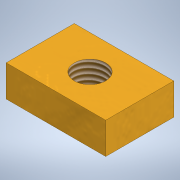
# Autodesk Inventor part: Part26
Saved by Autodesk Inventor 2020 (Build 240168000, 168)
## iProperties
Created: 2021-10-14
Part Number: Part26
Material: Brass, Soft Yellow, Welded
Document SubType Name: Modeling
Designer: simon.erikssonwestl
Density: 8.5 g/cm^3
Appearance: Weld - Brass
Author: simon.erikssonwestl
Autodesk Inventor part; units mm, degrees
ref_plane "YZ Plane" through (0, 0, 0) normal (1, 0, 0) x (0, 1, 0)
ref_plane "XZ Plane" through (0, 0, 0) normal (0, 1, 0) x (-1, 0, 0)
ref_plane "XY Plane" through (0, 0, 0) normal (0, 0, 1) x (1, 0, 0)
sketch "Sketch1" plane through (0, 0, 0) normal (0, 1, 0) x (-1, 0, 0)
  line L0 (4.75, 3.25) -> (-4.75, 3.25)
  line L1 (-4.75, 3.25) -> (-4.75, -3.25)
  line L2 (-4.75, -3.25) -> (4.75, -3.25)
  line L3 (4.75, -3.25) -> (4.75, 3.25)
  line L4 (4.75, 3.25) -> (-4.75, -3.25) construction
  line L5 (-4.75, 3.25) -> (4.75, -3.25) construction
  circle A0 centre (0, 0) radius 1.5
  dimension "d0" = 9.5
  dimension "d1" = 6.5
  dimension "d2" = 3
  constraints: 12 end point, 2 midpoint, 2 parallel, 1 centre point, 1 coincident, 1 horizontal, 1 perpendicular
  measures "d0" distance of L2.end L1.end
  measures "d1" distance of L1.end L0.end
  measures "d2" diameter of A0
extrude "Extrusion1" add sketch "Sketch1" along normal blind 3
thread "Thread1" size "M3x0.5" class "6H" standard "ANSI Metric M Profile" full length
body "Solid1"
